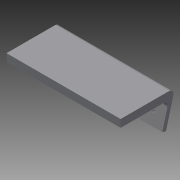
# Autodesk Inventor part: cubierta-edison
Saved by Autodesk Inventor 2015 SP1 (Build 190203100, 203)
## iProperties
Created: 2015-07-25
Part Number: cubierta-edison
Material: Genérico
Document SubType Name: Modeling
Designer: Javier
Density: 1 g/cm^3
Appearance: Valor por defecto
Author: Javier
Autodesk Inventor part; units mm, degrees
ref_plane "YZ Plane" through (0, 0, 0) normal (1, 0, 0) x (0, 1, 0)
ref_plane "XZ Plane" through (0, 0, 0) normal (0, 1, 0) x (-1, 0, 0)
ref_plane "XY Plane" through (0, 0, 0) normal (0, 0, 1) x (1, 0, 0)
sketch "Boceto1" plane through (0, 0, 0) normal (0, 0, 1) x (1, 0, 0)
  line L0 (-75, -35) -> (75, -35)
  line L1 (75, -35) -> (75, 35)
  line L2 (75, 35) -> (-75, 35)
  line L3 (-75, 35) -> (-75, -35)
  line L4 (-75, -35) -> (75, 35) construction
  line L5 (75, -35) -> (-75, 35) construction
  point P0 (0, 0)
  dimension "d0" = 150
  dimension "d1" = 70
  constraints: 12 end point, 2 midpoint, 2 parallel, 1 horizontal, 1 perpendicular
  measures "d0" distance of L2.end L1.end
  measures "d1" distance of L1.end L0.end
extrude "Extrusión1" add sketch "Boceto1" along normal blind 5
sketch "Boceto2" plane through (75, -35, 0) normal (1, 0, 0) x (0, 0, -1)
  line L0 (0, 0) -> (0, 70) projected
  line L1 (0, 70) -> (-5, 70) projected
  line L2 (-5, 0) -> (-5, 70) projected
  line L3 (0, 0) -> (-5, 0) projected
  line L4 (0, 70) -> (38.637, 59.6472)
  line L5 (0, 70) -> (40, 70) construction
  line L6 (38.637, 59.6472) -> (37.3429, 54.8176)
  line L7 (37.3429, 54.8176) -> (0, 64.8236)
  line L8 (0, 0) -> (0, 70) projected
  point P0 (0, 35)
  dimension "d4" = 40
  dimension "d5" = 15
  dimension "d6" = 5
  constraints: 8 end point, 1 equal length, 1 horizontal, 1 parallel, 1 perpendicular, 1 point on line
  measures "d4" distance of L0.end L4.end
  measures "d5" angle of L4 L5
  measures "d6" distance of L4.end L6.end
extrude "Extrusión2" add sketch "Boceto2" against normal up to surface (150 mm away) contours L0 L4 L6 L7
sketch "Boceto3" plane through (-75, -35, 0) normal (0, -1, 0) x (1, 0, 0)
  line L0 (0, 0) -> (150, 0) projected
  line L1 (150, 0) -> (150, 5) projected
  line L2 (0, 5) -> (150, 5) projected
  line L3 (0, 0) -> (0, 5) projected
  line L4 (150, 0) -> (150, -5)
  line L5 (150, -38.637) -> (150, 0) projected
  line L6 (150, -5) -> (145, -5)
  line L7 (145, -5) -> (145, 0)
  line L8 (0, 0) -> (0, -37.3429) projected
  line L9 (0, 0) -> (0, -5)
  line L10 (0, -5) -> (5, -5)
  line L11 (5, -5) -> (5, 0)
  line L12 (0, 0) -> (150, 0) projected
  point P0 (75, 0)
  dimension "d9" = 5
  dimension "d10" = 5
  dimension "d14" = 5
  dimension "d15" = 5
  constraints: 12 end point, 4 point on line, 3 perpendicular, 1 parallel
  measures "d9" distance of L0.end L4.end
  measures "d10" distance of L4.end L6.end
  measures "d14" distance of L0.start L9.end
  measures "d15" distance of L9.end L10.end
extrude "Extrusión3" add sketch "Boceto3" against normal up to surface contours L0 L11 L10 L8 | L0 L4 L6 L7 surface through (75, 19.8176, -37.3429) normal (0, -0.9659258, 0.258819)
sketch "Boceto4" plane through (-70, -35, 0) normal (1, 0, 0) x (0, 0, -1)
  line L0 (0, 64.8236) -> (5, 63.4839) projected
  line L1 (0, 0) -> (0, 64.8236) projected
  line L2 (5, 0) -> (0, 0) projected
  line L3 (5, 0) -> (5, 63.4839) projected
  line L4 (0, 0) -> (5, 0)
  line L5 (5, 0) -> (5, 5)
  line L6 (5, 0) -> (5, 63.4839) projected
  line L7 (5, 5) -> (0, 5)
  point P0 (0, 35)
  dimension "d16" = 5
  constraints: 6 end point, 2 perpendicular, 2 point on line
  measures "d16" distance of L2.start L5.end
extrude "Extrusión4" add sketch "Boceto4" along normal up to surface (140 mm away) contours L7 L3 L2 L1
fillet "Empalme1" radius 6 5 edges at (72.5, 28.4839, -5) (-72.5, 28.4839, -5) (0, 29.8236, 0) (0, 35, 5) (0, 35, 0)
sketch "Boceto5" plane through (-75, 24.6472, -38.637) normal (0, 0.9659258, -0.258819) x (1, 0, 0)
  line L0 (150, -37.357) -> (0, -37.357) projected
  line L1 (150, 0) -> (150, -37.357) projected
  line L2 (150, 0) -> (0, 0) projected
  line L3 (0, 0) -> (0, -37.357) projected
  line L4 (150, 0) -> (150, -15)
  line L5 (150, -15) -> (135, -15)
  line L6 (150, -15) -> (165, -15) construction
  circle A0 centre (135, -15) radius 1.5
  line L7 (135, -15) -> (35, -15)
  circle A1 centre (35, -15) radius 1.5
  point P0 (75, -30.9413)
  dimension "d20" = 15
  dimension "d21" = 15
  dimension "d22" = 180
  dimension "d23" = 3
  dimension "d24" = 100
  dimension "d25" = 3
  constraints: 8 end point, 2 centre point, 2 coincident, 2 horizontal, 1 collinear, 1 perpendicular, 1 vertical
  measures "d20" distance of L1.start L4.end
  measures "d21" distance of L4.end L5.end
  measures "d22" angle of L5 L6
  measures "d23" diameter of A0
  measures "d24" distance of L7.start L7.end
  measures "d25" diameter of A1
extrude "Extrusión5" cut sketch "Boceto5" against normal blind 5 contours A0 L7 L5 | L5 L7 A0 | A1
